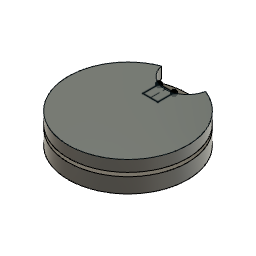
locking ring solids (Autodesk Fusion 360 design; units mm, degrees)
Autodesk Fusion 360 part; units mm, degrees
note: some values were not read from the file. Set by a fixed rule: which sketch regions a step uses.
sketch "Base" plane through (0, 0, 0) normal (0, 1, 0) x (1, 0, 0)
  circle A0 centre (0, 0) radius 25.4
  dimension "d1" = 50.8
  constraint coincident A0.centre origin
  measures "d1" diameter of A0
extrude "Extrude1" add sketch "Base" along normal blind 12.7 makes body 1
sketch "Relief" plane through (0, 12.7, 0) normal (0, 1, 0) x (-1, 0, 0)
  circle A0 centre (0, 0) radius 25.4
  circle A1 centre (0, -25.4) radius 9.525
  dimension "d4" = 19.05
  constraint coincident A0 A1.centre
  constraint vertical A0.centre A1.centre
  measures "d4" diameter of A1
extrude "Extrude2" cut sketch "Relief" against normal blind 6.35 contours A0 A1 | A0 A1 picked at (1.7493, -22.2335) picked at (2.3346, -28.2419) bodies 1
sketch "Boss Ref" plane through (0, 12.7, 0) normal (0, 1, 0) x (-1, 0, 0)
  arc A0 (9.3561, -23.6141) -> (-9.3561, -23.6141) centre (0, -25.4) ccw
  arc A1 (9.3561, -23.6141) -> (-9.3561, -23.6141) centre (0, 0) ccw
  circle A2 centre (0, -10.795) radius 4.7625
  circle A3 centre (0, -10.795) radius 2.5527
  dimension "d7" = 9.525
  dimension "d8" = 10.795
  dimension "d9" = 5.1054
  constraint vertical A1.centre A2.centre
  constraint concentric A2 A3
  measures "d7" diameter of A2
  measures "d8" distance of A1.centre A2.centre
  measures "d9" diameter of A3
sketch "Revolve Cut1" plane through (0, 0, 0) normal (1, 0, 0) x (0, 0, -1)
  line L0 (25.4, 0) -> (25.4, 6.35)
  line L1 (-25.4, 12.7) -> (-25.4, 0)
  line L2 (15.875, 6.35) -> (23.6141, 6.35)
  line L3 (25.4, 6.35) -> (22.225, 6.35)
  line L4 (22.225, 7.9375) -> (25.4, 7.9375)
  line L5 (25.4, 7.9375) -> (25.4, 6.35)
  line L6 (22.225, 7.9375) -> (22.225, 6.35)
  dimension "d12" = 3.175
  dimension "d13" = 1.5875
  constraint coincident L0.end L3.start
  constraint coincident L2 L3.end
  constraint perpendicular L0 L3
  constraint perpendicular L0 L4
  constraint perpendicular L3 L5
  constraint perpendicular L2 L6
  measures "d12" distance of L0.end L3.end
  measures "d13" distance of L4.end L0.end
revolve "Revolve1" cut sketch "Revolve Cut1" angle 360 about axis through (0, 1.75, 0) along (0, 1, 0) bodies 1
sketch "Sketch5" plane through (0, 12.7, 0) normal (0, 1, 0) x (-1, 0, 0)
  arc A0 (9.3561, -23.6141) -> (-9.3561, -23.6141) centre (0, -25.4) ccw
  arc A1 (9.3561, -23.6141) -> (-9.3561, -23.6141) centre (0, 0) ccw
  arc A2 (-8.2489, -20.6375) -> (-9.3561, -23.6141) centre (0, -25.4) ccw
  arc A3 (9.3561, -23.6141) -> (-9.3561, -23.6141) centre (0, 0) ccw
  arc A4 (9.3561, -23.6141) -> (8.2489, -20.6375) centre (0, -25.4) ccw
  arc A5 (8.2489, -20.6375) -> (-8.2489, -20.6375) centre (0, 0) ccw
  line L0 (0, -15.875) -> (-6.35, -9.525)
  line L1 (0, -15.875) -> (6.35, -9.525)
  line L2 (6.35, -9.525) -> (-6.35, -9.525)
  line L3 (0, -9.525) -> (0, -15.875) construction
  line L4 (6.35, -3.175) -> (-6.35, -3.175)
  line L5 (6.35, -9.525) -> (6.35, -3.175)
  line L6 (-6.35, -9.525) -> (-6.35, -3.175)
  line L7 (-6.35, -3.175) -> (-12.7, -3.175)
  line L8 (-12.7, -3.175) -> (-6.35, -9.525)
  line L9 (6.35, -9.525) -> (12.7, -3.175)
  line L10 (12.7, -3.175) -> (6.35, -3.175)
  dimension "d15" = 6.35
  dimension "d16" = 45
  dimension "d17" = 6.35
  constraint midpoint A0 L0.start
  constraint horizontal L2
  constraint midpoint L2 L3.start
  constraint perpendicular L2 L3
  constraint parallel L2 L4
  constraint equal L2 L4
  constraint vertical L1.end L4.start
  constraint perpendicular L6 L7
  constraint collinear L0 L8
  constraint parallel L1 L9
  constraint collinear L4 L10
  measures "d15" distance of L0.start L2
  measures "d16" angle of L0 L3
  measures "d17" distance of L2 L4
ref_plane "WorkPlane1" through (0, 0, -23.6141) normal (0, 0, 1) x (1, 0, 0)
sketch "Loft Profile 2" plane through (0, 12.7, 0) normal (0, 1, 0) x (-1, 0, 0)
  arc A0 (9.3561, -23.6141) -> (-9.3561, -23.6141) centre (0, -25.4) ccw
  arc A1 (9.3561, -23.6141) -> (-9.3561, -23.6141) centre (0, 0) ccw
  line L0 (4.7625, 8.255) -> (-4.7625, 8.255)
  arc A2 (-4.7625, 8.255) -> (-4.7625, -8.255) centre (-4.7625, 0) ccw
  line L1 (-4.7625, -8.255) -> (4.7625, -8.255)
  arc A3 (4.7625, -8.255) -> (4.7625, 8.255) centre (4.7625, 0) ccw
  line L2 (4.7625, 0) -> (-4.7625, 0) construction
  dimension "d19" = 9.525
  dimension "d20" = 8.255
  constraint tangent L0 A2
  constraint tangent A2 L1
  constraint parallel L0 L1
  constraint tangent L1 A3
  constraint tangent L0 A3
  constraint horizontal L2
  constraint coincident A1.centre origin
  constraint midpoint L2 A1.centre
  measures "d19" distance of A3.centre A2.centre
  measures "d20" radius of A2
sketch "Loft Profile 1" plane through (0, 0, 0) normal (0, -1, 0) x (1, 0, 0)
  circle A0 centre (0, 0) radius 25.4
  circle A1 centre (0, 0) radius 6.35
  dimension "d21" = 12.7
  constraint concentric A0 A1
  measures "d21" diameter of A1
sketch "Sweep Profile" plane through (0, 0, 0) normal (0, -1, 0) x (1, 0, 0)
  circle A0 centre (0, 0) radius 25.4
  circle A1 centre (0, 0) radius 19.05
  dimension "d22" = 38.1
  constraint coincident A0.centre A1.centre
  measures "d22" diameter of A1
sketch "Sweep Path" plane through (0, 0, 0) normal (0, 0, 1) x (1, 0, 0)
  line L0 (0, 0) -> (0, -63.5)
  arc A0 (0, -63.5) -> (50.1381, -135.1046) centre (76.2, -63.5) ccw
  line L1 (50.1381, -135.1046) -> (169.479, -178.5411)
  dimension "d23" = 76.2
  dimension "d24" = 63.5
  dimension "d25" = 127
  dimension "d26" = 110
  constraint coincident L0.start origin
  constraint vertical L0
  constraint tangent L0 A0
  constraint tangent A0 L1
  measures "d23" radius of A0
  measures "d24" distance of L0.start L0.end
  measures "d25" distance of A0.end L1.end
  measures "d26" angle of L0 L1
sketch "Hole Loc1" plane through (0, 12.7, 0) normal (0, 1, 0) x (-1, 0, 0)
  arc A0 (9.3561, -23.6141) -> (-9.3561, -23.6141) centre (0, -25.4) ccw
  arc A1 (9.3561, -23.6141) -> (-9.3561, -23.6141) centre (0, 0) ccw
  line L0 (0, 0) -> (0, -15.875) construction
  line L1 (0, 0) -> (-11.2253, -11.2253) construction
  point P0 (-11.2253, -11.2253)
  point P1 (11.2253, -11.2253)
  point P2 (11.2253, 11.2253)
  point P3 (-11.2253, 11.2253)
  dimension "d27" = 45
  dimension "d29" = 360
  constraint midpoint A0 L0.end
  constraint equal L0 L1
  constraint coincident A1.centre L0.start
  constraint coincident P0 L1.end
  measures "d27" angle of L0 L1
sketch "Extrude" plane through (0, 12.7, 0) normal (0, 1, 0) x (-1, 0, 0)
  arc A0 (9.3561, -23.6141) -> (-9.3561, -23.6141) centre (0, -25.4) ccw
  arc A1 (9.3561, -23.6141) -> (-9.3561, -23.6141) centre (0, 0) ccw
  line L0 (3.175, -16.4197) -> (-3.175, -16.4197)
  line L1 (-3.175, -16.4197) -> (-3.175, -9.525)
  line L2 (-3.175, -9.525) -> (3.175, -9.525)
  line L3 (3.175, -9.525) -> (3.175, -16.4197)
  line L4 (0, -9.525) -> (0, -15.875) construction
  dimension "d30" = 6.35
  dimension "d31" = 6.35
  constraint horizontal L0
  constraint vertical L1
  constraint horizontal L2
  constraint vertical L3
  constraint coincident A0 L0.start
  constraint coincident A0 L0.end
  constraint midpoint L2 L4.start
  constraint midpoint A0 L4.end
  measures "d30" distance of L0.start L0.end
  measures "d31" distance of L4.start L4.end
sketch "Revolve Cut2" plane through (0, 0, 0) normal (1, 0, 0) x (0, 0, -1)
  line L0 (25.4, 3.175) -> (22.225, 3.175)
  line L1 (22.225, 3.175) -> (22.225, 1.5875)
  line L2 (22.225, 1.5875) -> (25.4, 1.5875)
  line L3 (25.4, 1.5875) -> (25.4, 3.175)
  line L4 (25.4, 0) -> (25.4, 6.35)
  line L5 (22.225, 7.9375) -> (22.225, 6.35)
  constraint horizontal L0
  constraint vertical L1
  constraint horizontal L2
  constraint vertical L3
  constraint midpoint L0.start L4
  constraint collinear L1 L5
  constraint equal L1 L5
sketch "New Body" plane through (0, 12.7, 0) normal (0, 1, 0) x (-1, 0, 0)
  arc A0 (-4.7625, 8.255) -> (-4.7625, -8.255) centre (-4.7625, 0) ccw
  line L0 (-4.7625, -8.255) -> (4.7625, -8.255)
  arc A1 (4.7625, -8.255) -> (4.7625, 8.255) centre (4.7625, 0) ccw
  line L1 (4.7625, 8.255) -> (-4.7625, 8.255)
  line L2 (-4.7625, -9.525) -> (4.7625, -9.525)
  arc A2 (4.7625, -9.525) -> (4.7625, 9.525) centre (4.7625, 0) ccw
  line L3 (4.7625, 9.525) -> (-4.7625, 9.525)
  arc A3 (-4.7625, 9.525) -> (-4.7625, -9.525) centre (-4.7625, 0) ccw
  dimension "d32" = 1.27
extrude "Extrude4" add sketch "New Body" along normal blind 6.35 separate body contours A0 L0 A1 L1 | L2 A2 L3 A3 makes body 2
sketch "Sweep Guide" plane through (0, 0, 0) normal (0, 0, 1) x (1, 0, 0)
  line L0 (-25.4, 0) -> (25.4, 0)
  line L1 (25.4, 0) -> (25.4, -63.5)
  arc A0 (25.4, -63.5) -> (76.2, -114.3) centre (76.2, -63.5) ccw
  line L2 (76.2, -114.3) -> (169.479, -114.3)
  point P0 (76.2, -63.5)
  point P1 (169.479, -178.5411)
  constraint coincident L0.end L1.start
  constraint perpendicular L0 L1
  constraint tangent L1 A0
  constraint perpendicular L1 L2
  constraint tangent A0 L2
  constraint coincident P0 A0.centre
  constraint vertical L2.end P1
hidden bodies 2
equation "d17 = d15"
named bodies: "Locking Ring", "Inlet"
